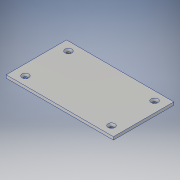
# Autodesk Inventor part: Piston Feed Surface
Saved by Autodesk Inventor 2018 (Build 220112000, 112)
## iProperties
Created: 2017-09-25
Part Number: Piston Feed Surface
Material: Aluminum 6061
Document SubType Name: Modeling
Designer: Gabriel Smolnycki
Density: 2.7 g/cm^3
Appearance: Aluminum - Flat
Author: Gabriel Smolnycki
Autodesk Inventor part; units mm, degrees
ref_plane "YZ Plane" through (0, 0, 0) normal (1, 0, 0) x (0, 1, 0)
ref_plane "XZ Plane" through (0, 0, 0) normal (0, 1, 0) x (-1, 0, 0)
ref_plane "XY Plane" through (0, 0, 0) normal (0, 0, 1) x (1, 0, 0)
sketch "Sketch1" plane through (0, 0, 0) normal (0, 1, 0) x (-1, 0, 0)
  line L0 (-74.75, 42.075) -> (74.75, 42.075)
  line L1 (74.75, 42.075) -> (74.75, -42.075)
  line L2 (74.75, -42.075) -> (-74.75, -42.075)
  line L3 (-74.75, -42.075) -> (-74.75, 42.075)
  line L4 (-74.75, 42.075) -> (74.75, -42.075) construction
  line L5 (74.75, 42.075) -> (-74.75, -42.075) construction
  point P0 (0, 0)
  dimension "d0" = 149.5
  dimension "d1" = 84.15
  constraints: 12 end point, 2 midpoint, 2 parallel, 1 horizontal, 1 perpendicular
  measures "d0" distance of L1.end L2.end
  measures "d1" distance of L0.end L1.end
extrude "Extrusion1" add sketch "Sketch1" along normal blind 4.064
sketch "Sketch2" plane through (0, 4.064, 0) normal (0, 1, 0) x (1, 0, 0)
  point P0 (0, 0)
  point P1 (-60, 30)
  point P2 (60, 30)
  point P3 (-60, -30)
  point P4 (60, -30)
  dimension "d4" = 60
  dimension "d5" = 30
  dimension "d6" = 60
  dimension "d7" = 30
  dimension "d8" = 30
  dimension "d9" = 60
  dimension "d10" = 30
  dimension "d11" = 60
  measures "d4" horizontal distance of point (-60, 30) point (0, 0)
  measures "d5" vertical distance of point (0, 0) point (-60, 30)
  measures "d6" horizontal distance of point (60, 30) point (0, 0)
  measures "d7" vertical distance of point (0, 0) point (60, 30)
  measures "d8" vertical distance of point (-60, -30) point (0, 0)
  measures "d9" horizontal distance of point (-60, -30) point (0, 0)
  measures "d10" vertical distance of point (60, -30) point (0, 0)
  measures "d11" horizontal distance of point (60, -30) point (0, 0)
hole "Hole1" at (-60, 4.064, -30) at (60, 4.064, -30) at (-60, 4.064, 30) at (60, 4.064, 30) direction (0, -1, 0) diameter 4.5 end through all countersink diameter 9.4 countersink angle 90
body "Solid1"
